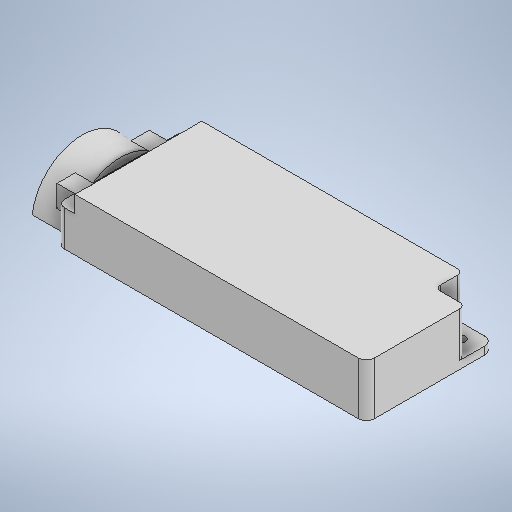
# Autodesk Inventor part: case_top
Saved by Autodesk Inventor 2025.2 (Build 292293000, 293)
## iProperties
Created: 2025-03-24
Part Number: case_top
Material: Generic
Document SubType Name: Modeling
Designer: Acer
Density: 1 g/cm^3
Appearance: Default
Author: Acer
Autodesk Inventor part; units mm, degrees
ref_plane "YZ Plane" through (0, 0, 0) normal (1, 0, 0) x (0, 1, 0)
ref_plane "XZ Plane" through (0, 0, 0) normal (0, 1, 0) x (-1, 0, 0)
ref_plane "XY Plane" through (0, 0, 0) normal (0, 0, 1) x (1, 0, 0)
sketch "Sketch1" plane through (0, 0, 0) normal (0, 1, 0) x (-1, 0, 0)
  line L0 (-55.3, 22.7) -> (55.3, 22.7)
  line L1 (55.3, 22.7) -> (55.3, -22.7)
  line L2 (55.3, -22.7) -> (-55.3, -22.7)
  line L3 (-55.3, -22.7) -> (-55.3, 22.7)
  line L4 (-55.3, 22.7) -> (55.3, -22.7) construction
  line L5 (55.3, 22.7) -> (-55.3, -22.7) construction
  point P0 (0, 0)
  dimension "d0" = 110.6
  dimension "d1" = 45.4
  constraints: 12 end point, 2 midpoint, 2 parallel, 1 horizontal, 1 perpendicular
  measures "d0" distance of L1.end L2.end
  measures "d1" distance of L0.end L1.end
extrude "Extrusion1" add sketch "Sketch1" along normal blind 18.8
sketch "Sketch2" plane through (0, 18.8, 0) normal (0, 1, 0) x (1, 0, 0)
  line L0 (55.3, -22.7) -> (55.3, 22.7) projected
  line L1 (55.3, 22.7) -> (45.3, 22.7)
  line L2 (45.3, 20.7) -> (45.3, 14.7)
  line L3 (47.3, 12.7) -> (53.3, 12.7)
  line L4 (55.3, 12.7) -> (55.3, 22.7)
  arc A0 (45.3, 14.7) -> (47.3, 12.7) centre (47.3, 14.7) ccw
  line L5 (43.3, 22.7) -> (43.3, 22.7)
  line L6 (55.3, 22.7) -> (-55.3, 22.7) projected
  line L7 (55.3, 10.7) -> (55.3, 10.7)
  arc A1 (55.3, 10.7) -> (53.3, 12.7) centre (53.3, 10.7) ccw
  arc A2 (45.3, 20.7) -> (43.3, 22.7) centre (43.3, 20.7) ccw
  point P0 (0, 0)
  point P1 (45.3, 12.7)
  dimension "d4" = 10
  dimension "d5" = 10
  dimension "d6" = 2
  dimension "d7" = 2
  dimension "d8" = 2
  dimension "d9" = 2
  constraints: 12 end point, 8 point on line, 6 point on circle, 6 tangent, 3 centre point, 2 parallel, 1 equal radius, 1 horizontal, 1 perpendicular
  measures "d4" distance of L4.start point (45.3, 12.7)
  measures "d5" distance of point (45.3, 12.7) L1.end
  measures "d6" radius of A0
  measures "d7" distance of L1.end L5.end
  measures "d8" distance of L4.start L7.end
  measures "d9" radius of A1
extrude "Extrusion2" cut sketch "Sketch2" against normal blind 16
sketch "Sketch4" plane through (0, 2.8, 0) normal (0, 1, 0) x (1, 0, 0)
  line L0 (55.3, -22.7) -> (55.3, 22.7) projected
  line L1 (55.3, 19.7) -> (55.3, 19.7)
  line L2 (52.3, 22.7) -> (52.3, 22.7)
  line L3 (43.3, 22.7) -> (55.3, 22.7) projected
  arc A0 (55.3, 19.7) -> (52.3, 22.7) centre (52.3, 19.7) ccw
  point P0 (0, 0)
  dimension "d18" = 3
  dimension "d19" = 3
  dimension "d20" = 3
  constraints: 4 end point, 4 point on line, 2 point on circle, 2 tangent, 1 centre point
  measures "d18" distance of L0.end L1.end
  measures "d19" distance of L0.end L2.end
  measures "d20" radius of A0
extrude "Extrusion4" cut sketch "Sketch4" against normal blind 16
sketch "Sketch5" plane through (0, 18.8, 0) normal (0, 1, 0) x (1, 0, 0)
  line L0 (-55.3, -22.7) -> (55.3, -22.7) projected
  line L1 (52.3, -22.7) -> (52.3, -22.7)
  line L2 (52.3, -22.7) -> (55.3, -22.7)
  line L3 (55.3, -22.7) -> (55.3, 19.7) projected
  line L4 (55.3, -19.7) -> (55.3, -19.7)
  arc A0 (52.3, -22.7) -> (55.3, -19.7) centre (52.3, -19.7) ccw
  point P0 (0, 0)
  dimension "d23" = 3
  dimension "d24" = 3
  dimension "d25" = 3
  constraints: 6 end point, 4 point on line, 2 point on circle, 2 tangent, 1 centre point, 1 collinear
  measures "d23" distance of L0.end L1.end
  measures "d24" distance of L0.end L4.end
  measures "d25" radius of A0
extrude "Extrusion5" cut sketch "Sketch5" against normal blind 19
sketch "Sketch6" plane through (0, 18.8, 0) normal (0, 1, 0) x (1, 0, 0)
  line L0 (43.3, 22.7) -> (52.3, 22.7) projected
  line L1 (43.3, 22.7) -> (42.1, 22.7)
  line L2 (42.1, 22.7) -> (42.5, 22.7)
  line L3 (44.5, 20.7) -> (44.5, 14.7)
  line L4 (46.5, 12.7) -> (55.3, 12.7)
  arc A0 (44.5, 14.7) -> (46.5, 12.7) centre (46.5, 14.7) ccw
  arc A1 (44.5, 20.7) -> (42.5, 22.7) centre (42.5, 20.7) ccw
  line L5 (55.3, 12.7) -> (55.3, 22.7)
  line L6 (55.3, -19.7) -> (55.3, 19.7) projected
  line L7 (55.3, 22.7) -> (42.1, 22.7)
  point P0 (0, 0)
  point P1 (44.5, 22.7)
  point P2 (44.5, 12.7)
  dimension "d28" = 1.2
  dimension "d29" = 2.4
  dimension "d30" = 10
  dimension "d31" = 10.8
  dimension "d32" = 2
  dimension "d33" = 10
  constraints: 12 end point, 5 point on line, 4 point on circle, 4 tangent, 2 centre point, 2 collinear, 2 perpendicular, 1 equal radius
  measures "d28" distance of L0.start L1.end
  measures "d29" distance of L1.end point (44.5, 22.7)
  measures "d30" distance of point (44.5, 22.7) point (44.5, 12.7)
  measures "d31" distance of point (44.5, 12.7) L4.end
  measures "d32" radius of A0
  measures "d33" distance of L4.end L5.end
extrude "Extrusion6" cut sketch "Sketch6" against normal blind 16
sketch "Sketch7" plane through (0, 2.8, 0) normal (0, 1, 0) x (1, 0, 0)
  arc A0 (55.3, 19.7) -> (52.3, 22.7) centre (52.3, 19.7) ccw projected
  line L0 (52.3, 22.7) -> (48.9, 22.7)
  line L1 (42.5, 22.7) -> (52.3, 22.7) projected
  line L2 (48.9, 22.7) -> (48.9, 17.5)
  circle A1 centre (48.9, 17.5) radius 1.7
  point P0 (0, 0)
  dimension "d36" = 3.4
  dimension "d37" = 5.2
  dimension "d38" = 3.4
  constraints: 4 end point, 1 centre point, 1 coincident, 1 perpendicular, 1 point on line
  measures "d36" distance of L0.start L0.end
  measures "d37" distance of L0.end L2.end
  measures "d38" diameter of A1
extrude "Extrusion7" cut sketch "Sketch7" against normal blind 16
sketch "Sketch8" plane through (0, 18.8, 0) normal (0, 1, 0) x (1, 0, 0)
  line L0 (-55.3, 22.7) -> (-55.3, -22.7) projected
  line L1 (-52.8, 22.7) -> (-52.8, 22.7)
  line L2 (52.3, 22.7) -> (-55.3, 22.7) projected
  line L3 (-52.8, 22.7) -> (-55.3, 22.7)
  line L4 (-55.3, 20.2) -> (-55.3, 20.2)
  arc A0 (-52.8, 22.7) -> (-55.3, 20.2) centre (-52.8, 20.2) ccw
  point P0 (0, 0)
  dimension "d41" = 2.5
  dimension "d42" = 2.5
  dimension "d43" = 2.5
  constraints: 6 end point, 3 point on line, 2 point on circle, 2 tangent, 1 centre point, 1 collinear, 1 perpendicular
  measures "d41" distance of L0.start L1.end
  measures "d42" distance of L0.start L4.end
  measures "d43" radius of A0
extrude "Extrusion8" cut sketch "Sketch8" against normal blind 19
mirror "Mirror3" about plane through (0, 0, 0) normal (0, 0, 1) of "Extrusion8"
sketch "Sketch9" plane through (0, 18.8, 0) normal (0, 1, 0) x (1, 0, 0)
  arc A0 (-52.8, 22.7) -> (-55.3, 20.2) centre (-52.8, 20.2) ccw projected
  line L0 (-55.3, 20.2) -> (-55.3, 17.5)
  line L1 (-55.3, 20.2) -> (-55.3, -20.2) projected
  line L2 (-55.3, 17.5) -> (-55.3, 12.8)
  line L3 (-55.3, 12.8) -> (-55.3, 17.5)
  line L4 (-55.3, 17.5) -> (-50.6, 17.5)
  circle A1 centre (-50.6, 17.5) radius 1.7
  point P0 (0, 0)
  dimension "d46" = 2.7
  dimension "d47" = 4.7
  dimension "d48" = 4.7
  dimension "d49" = 3.4
  constraints: 8 end point, 2 point on line, 1 centre point, 1 coincident, 1 collinear, 1 perpendicular
  measures "d46" distance of L0.start L0.end
  measures "d47" distance of L0.end L2.end
  measures "d48" distance of L0.end L4.end
  measures "d49" diameter of A1
extrude "Extrusion9" cut sketch "Sketch9" against normal blind 20
mirror "Mirror4" about plane through (0, 0, 0) normal (0, 0, 1) of "Extrusion9"
sketch "Sketch10" plane through (-55.3, 0, -20.2) normal (-1, 0, 0) x (0, 0, 1)
  line L0 (20.2, 0) -> (20.2, -2.2)
  line L1 (0, 0) -> (40.4, 0) projected
  arc A0 (38.065, 0) -> (2.335, 0) centre (20.2, -2.2) ccw
  line L2 (2.335, 0) -> (38.065, 0)
  line L3 (39.4, 0) -> (36, 0) projected
  line L4 (2.335, 0) -> (38.065, 0)
  dimension "d52" = 2.2
  dimension "d54" = 18
  dimension "d55" = 35.7301
  constraints: 6 end point, 2 collinear, 2 point on circle, 1 centre point, 1 point on line, 1 vertical
  measures "d52" distance of L0.start L0.end
  measures "d54" radius of A0
  measures "d55" distance of L2.end L2.start
extrude "Extrusion10" add sketch "Sketch10" along normal blind 13.8
sketch "Sketch11" plane through (-55.3, 0, -20.2) normal (-1, 0, 0) x (0, 0, 1)
  line L0 (20.2, 0) -> (3.7, 0)
  line L1 (39.9, 0) -> (0.5, 0) projected
  line L2 (3.7, 0) -> (16.5, 0)
  line L3 (16.5, 0) -> (3.7, 0)
  line L4 (3.7, 0) -> (3.7, 12.8)
  line L5 (3.7, 12.8) -> (36.7, 12.8)
  line L6 (36.7, 12.8) -> (36.7, 0)
  dimension "d58" = 16.5
  dimension "d59" = 12.8
  dimension "d60" = 12.8
  dimension "d61" = 33
  dimension "d62" = 12.8
  constraints: 12 end point, 3 point on line, 2 perpendicular, 1 collinear
  measures "d58" distance of L0.start L0.end
  measures "d59" distance of L0.end L2.end
  measures "d60" distance of L0.end L4.end
  measures "d61" distance of L4.end L5.end
  measures "d62" distance of L5.end L6.end
extrude "Extrusion11" add sketch "Sketch11" along normal blind 6.3
sketch "Sketch12" plane through (-55.3, 0, -20.2) normal (-1, 0, 0) x (0, 0, 1)
  line L0 (42.9, 0) -> (42.9, 18.8) projected
  line L1 (42.9, 18.8) -> (-2.5, 18.8)
  line L2 (-2.5, 18.8) -> (-2.5, 12.8)
  line L3 (-2.5, 12.8) -> (42.9, 12.8)
  line L4 (42.9, 12.8) -> (42.9, 18.8)
  point P0 (20.2, 0)
  dimension "d65" = 45.4
  dimension "d66" = 6
  constraints: 8 end point, 2 parallel, 1 horizontal, 1 perpendicular
  measures "d65" distance of L3.end L2.end
  measures "d66" distance of L2.end L1.end
extrude "Extrusion12" cut sketch "Sketch12" against normal blind 6.3
body "Solid1"
